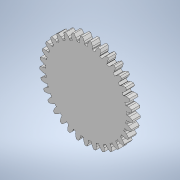
# Autodesk Inventor part: m1歯数33ギア3t
Saved by Autodesk Inventor 2020.2 (Build 242310000, 310)
## iProperties
Created: 2020-02-29
Part Number: m1歯数33ギア3t
Material: 一般
Document SubType Name: Modeling
Designer: aoyam
Density: 1 g/cm^3
Appearance: 既定
Author: aoyam
Autodesk Inventor part; units mm, degrees
ref_plane "YZ Plane" through (0, 0, 0) normal (1, 0, 0) x (0, 1, 0)
ref_plane "XZ Plane" through (0, 0, 0) normal (0, 1, 0) x (-1, 0, 0)
ref_plane "XY Plane" through (0, 0, 0) normal (0, 0, 1) x (1, 0, 0)
sketch "スケッチ1" plane through (0, 0, 0) normal (0, 0, 1) x (1, 0, 0)
  arc A0 (1.4847, 16.4043) -> (1.4561, 16.2027) centre (2.8638, 16.106) ccw
  arc A1 (1.672, 17.032) -> (1.4847, 16.4043) centre (5.2725, 15.6154) ccw
  arc A2 (2.2412, 18.1583) -> (1.672, 17.032) centre (7.8648, 14.6094) ccw
  arc A3 (0.4424, 16.2027) -> (0.4138, 16.4043) centre (-0.9654, 16.106) ccw
  arc A4 (0.4138, 16.4043) -> (0.2264, 17.032) centre (-3.3741, 15.6154) ccw
  arc A5 (0.2264, 17.032) -> (-0.3427, 18.1583) centre (-5.9663, 14.6094) ccw
  arc A6 (1.4478, 15.9479) -> (0.4507, 15.9479) centre (0.9492, 0.706) ccw
  arc A7 (-0.3427, 18.1583) -> (-1.085, 18.0874) centre (0.9492, 0.706) ccw
  line L0 (1.4478, 15.9479) -> (1.4561, 16.2027)
  line L1 (0.4507, 15.9479) -> (0.4424, 16.2027)
  arc A8 (-1.4959, 16.2219) -> (-1.4858, 16.0185) centre (-0.0852, 16.19) ccw
  arc A9 (-1.4458, 15.7668) -> (-2.4248, 15.5781) centre (0.9492, 0.706) ccw
  line L2 (-1.4458, 15.7668) -> (-1.4858, 16.0185)
  line L3 (-2.4248, 15.5781) -> (-2.4812, 15.8267)
  arc A10 (-2.4812, 15.8267) -> (-2.5474, 16.0192) centre (-3.8452, 15.4653) ccw
  arc A11 (-1.4307, 16.8737) -> (-1.4959, 16.2219) centre (2.3728, 16.1641) ccw
  arc A12 (-2.5474, 16.0192) -> (-2.8502, 16.6001) centre (-6.1176, 14.5278) ccw
  arc A13 (-3.6222, 17.5984) -> (-4.3377, 17.3883) centre (0.9492, 0.706) ccw
  arc A14 (-2.8502, 16.6001) -> (-3.6222, 17.5984) centre (-8.4726, 13.0493) ccw
  arc A15 (-1.085, 18.0874) -> (-1.4307, 16.8737) centre (5.1086, 15.6669) ccw
  arc A16 (-4.3881, 15.4788) -> (-4.3397, 15.281) centre (-2.9969, 15.7144) ccw
  arc A17 (-4.2528, 15.0414) -> (-5.1784, 14.6708) centre (0.9492, 0.706) ccw
  line L4 (-4.2528, 15.0414) -> (-4.3397, 15.281)
  line L5 (-5.1784, 14.6708) -> (-5.2808, 14.9042)
  arc A18 (-5.2808, 14.9042) -> (-5.3823, 15.0808) centre (-6.5518, 14.2913) ccw
  arc A19 (-4.4475, 16.1311) -> (-4.3881, 15.4788) centre (-0.5784, 16.1542) ccw
  arc A20 (-5.3823, 15.0808) -> (-5.7895, 15.5939) centre (-8.6056, 12.9406) ccw
  arc A21 (-6.7365, 16.4279) -> (-7.3993, 16.0863) centre (0.9492, 0.706) ccw
  arc A22 (-5.7895, 15.5939) -> (-6.7365, 16.4279) centre (-10.6383, 11.0432) ccw
  arc A23 (-4.3377, 17.3883) -> (-4.4475, 16.1311) centre (2.2021, 16.1837) ccw
  arc A24 (-7.0874, 14.2017) -> (-7.0025, 14.0167) centre (-5.7659, 14.6964) ccw
  arc A25 (-6.8717, 13.7978) -> (-7.7105, 13.2588) centre (0.9492, 0.706) ccw
  line L6 (-6.8717, 13.7978) -> (-7.0025, 14.0167)
  line L7 (-7.7105, 13.2588) -> (-7.8553, 13.4686)
  arc A26 (-7.8553, 13.4686) -> (-7.9883, 13.6227) centre (-8.9873, 12.6262) ccw
  arc A27 (-7.2692, 14.8311) -> (-7.0874, 14.2017) centre (-3.4744, 15.5859) ccw
  arc A28 (-7.9883, 13.6227) -> (-8.4853, 14.0495) centre (-10.7484, 10.9112) ccw
  arc A29 (-9.573, 14.6893) -> (-10.1591, 14.2284) centre (0.9492, 0.706) ccw
  arc A30 (-8.4853, 14.0495) -> (-9.573, 14.6893) centre (-12.3852, 8.6634) ccw
  arc A31 (-7.3993, 16.0863) -> (-7.2692, 14.8311) centre (-0.7497, 16.1411) ccw
  arc A32 (-9.4963, 12.4369) -> (-9.3778, 12.2712) centre (-8.2923, 13.1727) ccw
  arc A33 (-9.208, 12.0811) -> (-9.9296, 11.3931) centre (0.9492, 0.706) ccw
  line L8 (-9.208, 12.0811) -> (-9.3778, 12.2712)
  line L9 (-9.9296, 11.3931) -> (-10.1115, 11.5717)
  arc A34 (-10.1115, 11.5717) -> (-10.2713, 11.6979) centre (-11.0636, 10.5303) ccw
  arc A35 (-9.7938, 13.0204) -> (-9.4963, 12.4369) centre (-6.2105, 14.4799) ccw
  arc A36 (-10.2713, 11.6979) -> (-10.8401, 12.0229) centre (-12.4683, 8.513) ccw
  arc A37 (-12.0292, 12.4452) -> (-12.5175, 11.8817) centre (0.9492, 0.706) ccw
  arc A38 (-10.8401, 12.0229) -> (-12.0292, 12.4452) centre (-13.6502, 5.9961) ccw
  arc A39 (-10.1591, 14.2284) -> (-9.7938, 13.0204) centre (-3.6401, 15.5406) ccw
  arc A40 (-11.5276, 10.248) -> (-11.3799, 10.1078) centre (-10.4846, 11.1985) ccw
  arc A41 (-11.1772, 9.9532) -> (-11.7556, 9.1411) centre (0.9492, 0.706) ccw
  line L10 (-11.1772, 9.9532) -> (-11.3799, 10.1078)
  line L11 (-11.7556, 9.1411) -> (-11.968, 9.2821)
  arc A42 (-11.968, 9.2821) -> (-12.1487, 9.3758) centre (-12.7058, 8.0793) ccw
  arc A43 (-11.9302, 10.7648) -> (-11.5276, 10.248) centre (-8.6878, 12.876) ccw
  arc A44 (-12.1487, 9.3758) -> (-12.7687, 9.5872) centre (-13.7033, 5.8326) ccw
  arc A45 (-14.0164, 9.7769) -> (-14.3892, 9.1312) centre (0.9492, 0.706) ccw
  arc A46 (-12.7687, 9.5872) -> (-14.0164, 9.7769) centre (-14.3875, 3.1375) ccw
  arc A47 (-12.5175, 11.8817) -> (-11.9302, 10.7648) centre (-6.3647, 14.404) ccw
  arc A48 (-13.108, 7.7143) -> (-12.9364, 7.6046) centre (-12.2637, 8.845) ccw
  arc A49 (-12.7081, 7.4912) -> (-13.1223, 6.5843) centre (0.9492, 0.706) ccw
  line L12 (-12.7081, 7.4912) -> (-12.9364, 7.6046)
  line L13 (-13.1223, 6.5843) -> (-13.3576, 6.6825)
  arc A50 (-13.3576, 6.6825) -> (-13.5528, 6.7403) centre (-13.8544, 5.3618) ccw
  arc A51 (-13.6011, 8.1455) -> (-13.108, 7.7143) centre (-10.8168, 10.8322) ccw
  arc A52 (-13.5528, 6.7403) -> (-14.2016, 6.8306) centre (-14.4088, 2.967) ccw
  arc A53 (-15.4626, 6.7807) -> (-15.7065, 6.0761) centre (0.9492, 0.706) ccw
  arc A54 (-14.2016, 6.8306) -> (-15.4626, 6.7807) centre (-14.5705, 0.1911) ccw
  arc A55 (-14.3892, 9.1312) -> (-13.6011, 8.1455) centre (-8.8249, 12.7723) ccw
  arc A56 (-14.1803, 4.9274) -> (-13.9911, 4.8521) centre (-13.5652, 6.1973) ccw
  arc A57 (-13.7454, 4.7839) -> (-13.9805, 3.815) centre (0.9492, 0.706) ccw
  line L14 (-13.7454, 4.7839) -> (-13.9911, 4.8521)
  line L15 (-13.9805, 3.815) -> (-14.2301, 3.8669)
  arc A58 (-14.2301, 3.8669) -> (-14.4327, 3.8867) centre (-14.468, 2.4761) ccw
  arc A59 (-14.7461, 5.2574) -> (-14.1803, 4.9274) centre (-12.5206, 8.4225) ccw
  arc A60 (-14.4327, 3.8867) -> (-15.0869, 3.8526) centre (-14.5591, 0.0196) ccw
  arc A61 (-16.3156, 3.565) -> (-16.4218, 2.827) centre (0.9492, 0.706) ccw
  arc A62 (-15.0869, 3.8526) -> (-16.3156, 3.565) centre (-14.1926, -2.7368) ccw
  arc A63 (-15.7065, 6.0761) -> (-14.7461, 5.2574) centre (-10.9318, 10.7045) ccw
  arc A64 (-14.7057, 1.9878) -> (-14.5057, 1.9497) centre (-14.3422, 3.3512) ccw
  arc A65 (-14.2516, 1.9292) -> (-14.2991, 0.9333) centre (0.9492, 0.706) ccw
  line L16 (-14.2516, 1.9292) -> (-14.5057, 1.9497)
  line L17 (-14.2991, 0.9333) -> (-14.554, 0.9371)
  arc A66 (-14.554, 0.9371) -> (-14.7567, 0.9182) centre (-14.5244, -0.4736) ccw
  arc A67 (-15.3238, 2.2048) -> (-14.7057, 1.9878) centre (-13.7375, 5.7339) ccw
  arc A68 (-14.7567, 0.9182) -> (-15.3926, 0.7609) centre (-14.1489, -2.903) ccw
  arc A69 (-16.5447, 0.2459) -> (-16.5092, -0.4989) centre (0.9492, 0.706) ccw
  arc A70 (-15.3926, 0.7609) -> (-16.5447, 0.2459) centre (-13.2674, -5.5401) ccw
  arc A71 (-16.4218, 2.827) -> (-15.3238, 2.2048) centre (-12.6093, 8.2753) ccw
  arc A72 (-14.6654, -0.9981) -> (-14.4618, -0.9977) centre (-14.5664, 0.4095) ccw
  arc A73 (-14.2084, -0.9697) -> (-14.0665, -1.9566) centre (0.9492, 0.706) ccw
  line L18 (-14.2084, -0.9697) -> (-14.4618, -0.9977)
  line L19 (-14.0665, -1.9566) -> (-14.3175, -2.0011)
  arc A74 (-14.3175, -2.0011) -> (-14.513, -2.058) centre (-14.0215, -3.3807) ccw
  arc A75 (-15.3134, -0.902) -> (-14.6654, -0.9981) centre (-14.4236, 2.8635) ccw
  arc A76 (-14.513, -2.058) -> (-15.1077, -2.3328) centre (-13.1931, -5.6951) ccw
  arc A77 (-16.1415, -3.0565) -> (-15.9657, -3.7811) centre (0.9492, 0.706) ccw
  arc A78 (-15.1077, -2.3328) -> (-16.1415, -3.0565) centre (-11.8284, -8.1178) ccw
  arc A79 (-16.5092, -0.4989) -> (-15.3134, -0.902) centre (-13.7968, 5.5725) ccw
  arc A80 (-14.0607, -3.9224) -> (-13.8609, -3.8835) centre (-14.2299, -2.5215) ccw
  arc A81 (-13.6174, -3.808) -> (-13.2913, -4.7502) centre (0.9492, 0.706) ccw
  line L20 (-13.6174, -3.808) -> (-13.8609, -3.8835)
  line L21 (-13.2913, -4.7502) -> (-13.5293, -4.8414)
  arc A82 (-13.5293, -4.8414) -> (-13.7105, -4.9343) centre (-12.9775, -6.1401) ccw
  arc A83 (-14.7152, -3.9506) -> (-14.0607, -3.9224) centre (-14.5541, -0.0848) ccw
  arc A84 (-13.7105, -4.9343) -> (-14.2424, -5.3167) centre (-11.7261, -8.2559) ccw
  arc A85 (-15.1206, -6.223) -> (-14.8108, -6.9012) centre (0.9492, 0.706) ccw
  arc A86 (-14.2424, -5.3167) -> (-15.1206, -6.223) centre (-9.9276, -10.3765) ccw
  arc A87 (-15.9657, -3.7811) -> (-14.7152, -3.9506) centre (-14.4513, 2.6939) ccw
  arc A88 (-12.9135, -6.6794) -> (-12.7247, -6.6033) centre (-13.3448, -5.3359) ccw
  arc A89 (-12.4998, -6.4832) -> (-12.0013, -7.3466) centre (0.9492, 0.706) ccw
  line L22 (-12.4998, -6.4832) -> (-12.7247, -6.6033)
  line L23 (-12.0013, -7.3466) -> (-12.2178, -7.4812)
  arc A90 (-12.2178, -7.4812) -> (-12.3781, -7.6068) centre (-11.4302, -8.652) ccw
  arc A91 (-13.5508, -6.831) -> (-12.9135, -6.6794) centre (-14.1243, -3.0046) ccw
  arc A92 (-12.3781, -7.6068) -> (-12.828, -8.0829) centre (-9.801, -10.4928) ccw
  arc A93 (-13.5189, -9.139) -> (-13.0864, -9.7464) centre (0.9492, 0.706) ccw
  arc A94 (-12.828, -8.0829) -> (-13.5189, -9.139) centre (-7.6336, -12.2347) ccw
  arc A95 (-14.8108, -6.9012) -> (-13.5508, -6.831) centre (-14.5492, -0.2566) ccw
  arc A96 (-11.2653, -9.1695) -> (-11.0943, -9.0591) centre (-11.9431, -7.9319) ccw
  arc A97 (-10.8962, -8.8985) -> (-10.2433, -9.652) centre (0.9492, 0.706) ccw
  line L24 (-10.8962, -8.8985) -> (-11.0943, -9.0591)
  line L25 (-10.2433, -9.652) -> (-10.4304, -9.8252)
  arc A98 (-10.4304, -9.8252) -> (-10.5641, -9.9788) centre (-9.4355, -10.8258) ccw
  arc A99 (-11.8624, -9.4389) -> (-11.2653, -9.1695) centre (-13.1497, -5.7902) ccw
  arc A100 (-10.5641, -9.9788) -> (-10.9158, -10.5314) centre (-7.4873, -12.3249) ccw
  arc A101 (-11.3942, -11.6992) -> (-10.8546, -12.2137) centre (0.9492, 0.706) ccw
  arc A102 (-10.9158, -10.5314) -> (-11.3942, -11.6992) centre (-5.0295, -13.6252) ccw
  arc A103 (-13.0864, -9.7464) -> (-11.8624, -9.4389) centre (-14.0869, -3.1723) ccw
  arc A104 (-9.1756, -11.3026) -> (-9.0286, -11.1618) centre (-10.0754, -10.2156) ccw
  arc A105 (-8.8645, -10.9667) -> (-8.0808, -11.583) centre (0.9492, 0.706) ccw
  line L26 (-8.8645, -10.9667) -> (-9.0286, -11.1618)
  line L27 (-8.0808, -11.583) -> (-8.2317, -11.7885)
  arc A106 (-8.2317, -11.7885) -> (-8.3339, -11.9646) centre (-7.0654, -12.5827) ccw
  arc A107 (-9.7109, -11.6802) -> (-9.1756, -11.3026) centre (-11.6655, -8.341) ccw
  arc A108 (-8.3339, -11.9646) -> (-8.5746, -12.5738) centre (-4.8688, -13.686) ccw
  arc A109 (-8.8235, -13.811) -> (-8.1962, -14.2141) centre (0.9492, 0.706) ccw
  arc A110 (-8.5746, -12.5738) -> (-8.8235, -13.811) centre (-2.2092, -14.4977) ccw
  arc A111 (-10.8546, -12.2137) -> (-9.7109, -11.6802) centre (-13.0812, -5.9478) ccw
  arc A112 (-6.72, -13.0018) -> (-6.6022, -12.8357) centre (-7.8092, -12.1047) ccw
  arc A113 (-6.4781, -12.613) -> (-5.5919, -13.0699) centre (0.9492, 0.706) ccw
  line L28 (-6.4781, -12.613) -> (-6.6022, -12.8357)
  line L29 (-5.5919, -13.0699) -> (-5.7012, -13.3002)
  arc A114 (-5.7012, -13.3002) -> (-5.7682, -13.4925) centre (-4.4057, -13.8593) ccw
  arc A115 (-7.1742, -13.4738) -> (-6.72, -13.0018) centre (-9.7253, -10.5649) ccw
  arc A116 (-5.7682, -13.4925) -> (-5.8893, -14.1363) centre (-2.0399, -14.527) ccw
  arc A117 (-5.8995, -15.3982) -> (-5.2073, -15.6753) centre (0.9492, 0.706) ccw
  arc A118 (-5.8893, -14.1363) -> (-5.8995, -15.3982) centre (0.7251, -14.8207) ccw
  arc A119 (-8.1962, -14.2141) -> (-7.1742, -13.4738) centre (-11.5684, -8.4829) ccw
  arc A120 (-3.9872, -14.2055) -> (-3.903, -14.0201) centre (-5.2265, -13.5307) ccw
  arc A121 (-3.8232, -13.778) -> (-2.8666, -14.0589) centre (0.9492, 0.706) ccw
  line L30 (-3.8232, -13.778) -> (-3.903, -14.0201)
  line L31 (-2.8666, -14.0589) -> (-2.9303, -14.3057)
  arc A122 (-2.9303, -14.3057) -> (-2.9597, -14.5072) centre (-1.5524, -14.6095) ccw
  arc A123 (-4.3438, -14.755) -> (-3.9872, -14.2055) centre (-7.3994, -12.3814) ccw
  arc A124 (-2.9597, -14.5072) -> (-2.9568, -15.1622) centre (0.897, -14.8174) ccw
  arc A125 (-2.728, -16.4033) -> (-1.9958, -16.5444) centre (0.9492, 0.706) ccw
  arc A126 (-2.9568, -15.1622) -> (-2.728, -16.4033) centre (3.6676, -14.5825) ccw
  arc A127 (-5.2073, -15.6753) -> (-4.3438, -14.755) centre (-9.6032, -10.6858) ccw
  arc A128 (-1.076, -14.8702) -> (-1.0284, -14.6723) centre (-2.4205, -14.4422) ccw
  arc A129 (-0.9958, -14.4194) -> (-0.0033, -14.5142) centre (0.9492, 0.706) ccw
  line L32 (-0.9958, -14.4194) -> (-1.0284, -14.6723)
  line L33 (-0.0033, -14.5142) -> (-0.0193, -14.7686)
  arc A130 (-0.0193, -14.7686) -> (-0.01, -14.972) centre (1.3913, -14.8062) ccw
  arc A131 (-1.3222, -15.4773) -> (-1.076, -14.8702) centre (-4.7717, -13.7249) ccw
  arc A132 (-0.01, -14.972) -> (0.1169, -15.6147) centre (3.8357, -14.5468) ccw
  arc A133 (0.5764, -16.79) -> (1.3221, -16.79) centre (0.9492, 0.706) ccw
  arc A134 (0.1169, -15.6147) -> (0.5764, -16.79) centre (6.5119, -13.7917) ccw
  arc A135 (-1.9958, -16.5444) -> (-1.3222, -15.4773) centre (-7.2566, -12.477) ccw
  arc A136 (1.9085, -14.972) -> (1.9177, -14.7686) centre (0.5072, -14.8062) ccw
  arc A137 (1.9018, -14.5142) -> (2.8943, -14.4194) centre (0.9492, 0.706) ccw
  line L34 (1.9018, -14.5142) -> (1.9177, -14.7686)
  line L35 (2.8943, -14.4194) -> (2.9268, -14.6723)
  arc A138 (2.9268, -14.6723) -> (2.9744, -14.8702) centre (4.319, -14.4422) ccw
  arc A139 (1.7816, -15.6147) -> (1.9085, -14.972) centre (-1.9373, -14.5468) ccw
  arc A140 (2.9744, -14.8702) -> (3.2206, -15.4773) centre (6.6702, -13.7249) ccw
  arc A141 (3.8943, -16.5444) -> (4.6265, -16.4033) centre (0.9492, 0.706) ccw
  arc A142 (3.2206, -15.4773) -> (3.8943, -16.5444) centre (9.1551, -12.477) ccw
  arc A143 (1.3221, -16.79) -> (1.7816, -15.6147) centre (-4.6134, -13.7917) ccw
  arc A144 (4.8582, -14.5072) -> (4.8288, -14.3057) centre (3.4509, -14.6095) ccw
  arc A145 (4.765, -14.0589) -> (5.7217, -13.778) centre (0.9492, 0.706) ccw
  line L36 (4.765, -14.0589) -> (4.8288, -14.3057)
  line L37 (5.7217, -13.778) -> (5.8015, -14.0201)
  arc A146 (5.8015, -14.0201) -> (5.8857, -14.2055) centre (7.1249, -13.5307) ccw
  arc A147 (4.8553, -15.1622) -> (4.8582, -14.5072) centre (1.0015, -14.8174) ccw
  arc A148 (5.8857, -14.2055) -> (6.2423, -14.755) centre (9.2979, -12.3814) ccw
  arc A149 (7.1057, -15.6753) -> (7.798, -15.3982) centre (0.9492, 0.706) ccw
  arc A150 (6.2423, -14.755) -> (7.1057, -15.6753) centre (11.5017, -10.6858) ccw
  arc A151 (4.6265, -16.4033) -> (4.8553, -15.1622) centre (-1.7692, -14.5825) ccw
  arc A152 (7.6667, -13.4925) -> (7.5997, -13.3002) centre (6.3042, -13.8593) ccw
  arc A153 (7.4904, -13.0699) -> (8.3766, -12.613) centre (0.9492, 0.706) ccw
  line L38 (7.4904, -13.0699) -> (7.5997, -13.3002)
  line L39 (8.3766, -12.613) -> (8.5007, -12.8357)
  arc A154 (8.5007, -12.8357) -> (8.6185, -13.0018) centre (9.7077, -12.1047) ccw
  arc A155 (7.7878, -14.1363) -> (7.6667, -13.4925) centre (3.9384, -14.527) ccw
  arc A156 (8.6185, -13.0018) -> (9.0727, -13.4738) centre (11.6238, -10.5649) ccw
  arc A157 (10.0947, -14.2141) -> (10.7219, -13.811) centre (0.9492, 0.706) ccw
  arc A158 (9.0727, -13.4738) -> (10.0947, -14.2141) centre (13.4669, -8.4829) ccw
  arc A159 (7.798, -15.3982) -> (7.7878, -14.1363) centre (1.1733, -14.8207) ccw
  arc A160 (10.2324, -11.9646) -> (10.1302, -11.7885) centre (8.9639, -12.5827) ccw
  arc A161 (9.9793, -11.583) -> (10.763, -10.9667) centre (0.9492, 0.706) ccw
  line L40 (9.9793, -11.583) -> (10.1302, -11.7885)
  line L41 (10.763, -10.9667) -> (10.927, -11.1618)
  arc A162 (10.927, -11.1618) -> (11.0741, -11.3026) centre (11.9738, -10.2156) ccw
  arc A163 (10.4731, -12.5738) -> (10.2324, -11.9646) centre (6.7672, -13.686) ccw
  arc A164 (11.0741, -11.3026) -> (11.6094, -11.6802) centre (13.5639, -8.341) ccw
  arc A165 (12.7531, -12.2137) -> (13.2927, -11.6992) centre (0.9492, 0.706) ccw
  arc A166 (11.6094, -11.6802) -> (12.7531, -12.2137) centre (14.9797, -5.9478) ccw
  arc A167 (10.7219, -13.811) -> (10.4731, -12.5738) centre (4.1077, -14.4977) ccw
  arc A168 (12.4625, -9.9788) -> (12.3289, -9.8252) centre (11.334, -10.8258) ccw
  arc A169 (12.1418, -9.652) -> (12.7947, -8.8985) centre (0.9492, 0.706) ccw
  line L42 (12.1418, -9.652) -> (12.3289, -9.8252)
  line L43 (12.7947, -8.8985) -> (12.9927, -9.0591)
  arc A170 (12.9927, -9.0591) -> (13.1638, -9.1695) centre (13.8415, -7.9319) ccw
  arc A171 (12.8142, -10.5314) -> (12.4625, -9.9788) centre (9.3858, -12.3249) ccw
  arc A172 (13.1638, -9.1695) -> (13.7609, -9.4389) centre (15.0482, -5.7902) ccw
  arc A173 (14.9848, -9.7464) -> (15.4173, -9.139) centre (0.9492, 0.706) ccw
  arc A174 (13.7609, -9.4389) -> (14.9848, -9.7464) centre (15.9854, -3.1723) ccw
  arc A175 (13.2927, -11.6992) -> (12.8142, -10.5314) centre (6.928, -13.6252) ccw
  arc A176 (14.2766, -7.6068) -> (14.1163, -7.4812) centre (13.3287, -8.652) ccw
  arc A177 (13.8998, -7.3466) -> (14.3983, -6.4832) centre (0.9492, 0.706) ccw
  line L44 (13.8998, -7.3466) -> (14.1163, -7.4812)
  line L45 (14.3983, -6.4832) -> (14.6232, -6.6033)
  arc A178 (14.6232, -6.6033) -> (14.812, -6.6794) centre (15.2433, -5.3359) ccw
  arc A179 (14.7265, -8.0829) -> (14.2766, -7.6068) centre (11.6995, -10.4928) ccw
  arc A180 (14.812, -6.6794) -> (15.4493, -6.831) centre (16.0228, -3.0046) ccw
  arc A181 (16.7093, -6.9012) -> (17.0191, -6.223) centre (0.9492, 0.706) ccw
  arc A182 (15.4493, -6.831) -> (16.7093, -6.9012) centre (16.4477, -0.2566) ccw
  arc A183 (15.4173, -9.139) -> (14.7265, -8.0829) centre (9.5321, -12.2347) ccw
  arc A184 (15.609, -4.9343) -> (15.4278, -4.8414) centre (14.876, -6.1401) ccw
  arc A185 (15.1898, -4.7502) -> (15.5158, -3.808) centre (0.9492, 0.706) ccw
  line L46 (15.1898, -4.7502) -> (15.4278, -4.8414)
  line L47 (15.5158, -3.808) -> (15.7594, -3.8835)
  arc A186 (15.7594, -3.8835) -> (15.9592, -3.9224) centre (16.1284, -2.5215) ccw
  arc A187 (16.1409, -5.3167) -> (15.609, -4.9343) centre (13.6246, -8.2559) ccw
  arc A188 (15.9592, -3.9224) -> (16.6137, -3.9506) centre (16.4526, -0.0848) ccw
  arc A189 (17.8642, -3.7811) -> (18.04, -3.0565) centre (0.9492, 0.706) ccw
  arc A190 (16.6137, -3.9506) -> (17.8642, -3.7811) centre (16.3498, 2.6939) ccw
  arc A191 (17.0191, -6.223) -> (16.1409, -5.3167) centre (11.8261, -10.3765) ccw
  arc A192 (16.4115, -2.058) -> (16.216, -2.0011) centre (15.92, -3.3807) ccw
  arc A193 (15.965, -1.9566) -> (16.1069, -0.9697) centre (0.9492, 0.706) ccw
  line L48 (15.965, -1.9566) -> (16.216, -2.0011)
  line L49 (16.1069, -0.9697) -> (16.3603, -0.9977)
  arc A194 (16.3603, -0.9977) -> (16.5639, -0.9981) centre (16.4649, 0.4095) ccw
  arc A195 (17.0061, -2.3328) -> (16.4115, -2.058) centre (15.0916, -5.6951) ccw
  arc A196 (16.5639, -0.9981) -> (17.2119, -0.902) centre (16.3221, 2.8635) ccw
  arc A197 (18.4077, -0.4989) -> (18.4432, 0.2459) centre (0.9492, 0.706) ccw
  arc A198 (17.2119, -0.902) -> (18.4077, -0.4989) centre (15.6953, 5.5725) ccw
  arc A199 (18.04, -3.0565) -> (17.0061, -2.3328) centre (13.7269, -8.1178) ccw
  arc A200 (16.6552, 0.9182) -> (16.4524, 0.9371) centre (16.4229, -0.4736) ccw
  arc A201 (16.1975, 0.9333) -> (16.1501, 1.9292) centre (0.9492, 0.706) ccw
  line L50 (16.1975, 0.9333) -> (16.4524, 0.9371)
  line L51 (16.1501, 1.9292) -> (16.4042, 1.9497)
  arc A202 (16.4042, 1.9497) -> (16.6042, 1.9878) centre (16.2407, 3.3512) ccw
  arc A203 (17.2911, 0.7609) -> (16.6552, 0.9182) centre (16.0474, -2.903) ccw
  arc A204 (16.6042, 1.9878) -> (17.2223, 2.2048) centre (15.636, 5.7339) ccw
  arc A205 (18.3202, 2.827) -> (18.2141, 3.565) centre (0.9492, 0.706) ccw
  arc A206 (17.2223, 2.2048) -> (18.3202, 2.827) centre (14.5078, 8.2753) ccw
  arc A207 (18.4432, 0.2459) -> (17.2911, 0.7609) centre (15.1659, -5.5401) ccw
  arc A208 (16.3312, 3.8867) -> (16.1286, 3.8669) centre (16.3665, 2.4761) ccw
  arc A209 (15.879, 3.815) -> (15.6439, 4.7839) centre (0.9492, 0.706) ccw
  line L52 (15.879, 3.815) -> (16.1286, 3.8669)
  line L53 (15.6439, 4.7839) -> (15.8896, 4.8521)
  arc A210 (15.8896, 4.8521) -> (16.0787, 4.9274) centre (15.4637, 6.1973) ccw
  arc A211 (16.9854, 3.8526) -> (16.3312, 3.8867) centre (16.4576, 0.0196) ccw
  arc A212 (16.0787, 4.9274) -> (16.6446, 5.2574) centre (14.4191, 8.4225) ccw
  arc A213 (17.6049, 6.0761) -> (17.3611, 6.7807) centre (0.9492, 0.706) ccw
  arc A214 (16.6446, 5.2574) -> (17.6049, 6.0761) centre (12.8303, 10.7045) ccw
  arc A215 (18.2141, 3.565) -> (16.9854, 3.8526) centre (16.0911, -2.7368) ccw
  arc A216 (15.4513, 6.7403) -> (15.256, 6.6825) centre (15.7529, 5.3618) ccw
  arc A217 (15.0208, 6.5843) -> (14.6066, 7.4912) centre (0.9492, 0.706) ccw
  line L54 (15.0208, 6.5843) -> (15.256, 6.6825)
  line L55 (14.6066, 7.4912) -> (14.8349, 7.6046)
  arc A218 (14.8349, 7.6046) -> (15.0064, 7.7143) centre (14.1622, 8.845) ccw
  arc A219 (16.1001, 6.8306) -> (15.4513, 6.7403) centre (16.3072, 2.967) ccw
  arc A220 (15.0064, 7.7143) -> (15.4996, 8.1455) centre (12.7153, 10.8322) ccw
  arc A221 (16.2877, 9.1312) -> (15.9148, 9.7769) centre (0.9492, 0.706) ccw
  arc A222 (15.4996, 8.1455) -> (16.2877, 9.1312) centre (10.7233, 12.7723) ccw
  arc A223 (17.3611, 6.7807) -> (16.1001, 6.8306) centre (16.469, 0.1911) ccw
  arc A224 (14.0472, 9.3758) -> (13.8664, 9.2821) centre (14.6042, 8.0793) ccw
  arc A225 (13.6541, 9.1411) -> (13.0757, 9.9532) centre (0.9492, 0.706) ccw
  line L56 (13.6541, 9.1411) -> (13.8664, 9.2821)
  line L57 (13.0757, 9.9532) -> (13.2784, 10.1078)
  arc A226 (13.2784, 10.1078) -> (13.4261, 10.248) centre (12.3831, 11.1985) ccw
  arc A227 (14.6672, 9.5872) -> (14.0472, 9.3758) centre (15.6018, 5.8326) ccw
  arc A228 (13.4261, 10.248) -> (13.8287, 10.7648) centre (10.5863, 12.876) ccw
  arc A229 (14.416, 11.8817) -> (13.9277, 12.4452) centre (0.9492, 0.706) ccw
  arc A230 (13.8287, 10.7648) -> (14.416, 11.8817) centre (8.2632, 14.404) ccw
  arc A231 (15.9148, 9.7769) -> (14.6672, 9.5872) centre (16.286, 3.1375) ccw
  arc A232 (12.1698, 11.6979) -> (12.01, 11.5717) centre (12.9621, 10.5303) ccw
  arc A233 (11.8281, 11.3931) -> (11.1065, 12.0811) centre (0.9492, 0.706) ccw
  line L58 (11.8281, 11.3931) -> (12.01, 11.5717)
  line L59 (11.1065, 12.0811) -> (11.2763, 12.2712)
  arc A234 (11.2763, 12.2712) -> (11.3948, 12.4369) centre (10.1908, 13.1727) ccw
  arc A235 (12.7385, 12.0229) -> (12.1698, 11.6979) centre (14.3668, 8.513) ccw
  arc A236 (11.3948, 12.4369) -> (11.6923, 13.0204) centre (8.109, 14.4799) ccw
  arc A237 (12.0576, 14.2284) -> (11.4715, 14.6893) centre (0.9492, 0.706) ccw
  arc A238 (11.6923, 13.0204) -> (12.0576, 14.2284) centre (5.5386, 15.5406) ccw
  arc A239 (13.9277, 12.4452) -> (12.7385, 12.0229) centre (15.5487, 5.9961) ccw
  arc A240 (9.8868, 13.6227) -> (9.7537, 13.4686) centre (10.8857, 12.6262) ccw
  arc A241 (9.609, 13.2588) -> (8.7702, 13.7978) centre (0.9492, 0.706) ccw
  line L60 (9.609, 13.2588) -> (9.7537, 13.4686)
  line L61 (8.7702, 13.7978) -> (8.901, 14.0167)
  arc A242 (8.901, 14.0167) -> (8.9859, 14.2017) centre (7.6644, 14.6964) ccw
  arc A243 (10.3838, 14.0495) -> (9.8868, 13.6227) centre (12.6468, 10.9112) ccw
  arc A244 (8.9859, 14.2017) -> (9.1677, 14.8311) centre (5.3729, 15.5859) ccw
  arc A245 (9.2978, 16.0863) -> (8.635, 16.4279) centre (0.9492, 0.706) ccw
  arc A246 (9.1677, 14.8311) -> (9.2978, 16.0863) centre (2.6482, 16.1411) ccw
  arc A247 (11.4715, 14.6893) -> (10.3838, 14.0495) centre (14.2837, 8.6634) ccw
  arc A248 (7.2807, 15.0808) -> (7.1793, 14.9042) centre (8.4503, 14.2913) ccw
  arc A249 (7.0769, 14.6708) -> (6.1513, 15.0414) centre (0.9492, 0.706) ccw
  line L62 (7.0769, 14.6708) -> (7.1793, 14.9042)
  line L63 (6.1513, 15.0414) -> (6.2382, 15.281)
  arc A250 (6.2382, 15.281) -> (6.2866, 15.4788) centre (4.8954, 15.7144) ccw
  arc A251 (7.688, 15.5939) -> (7.2807, 15.0808) centre (10.5041, 12.9406) ccw
  arc A252 (6.2866, 15.4788) -> (6.346, 16.1311) centre (2.4769, 16.1542) ccw
  arc A253 (6.2362, 17.3883) -> (5.5207, 17.5984) centre (0.9492, 0.706) ccw
  arc A254 (6.346, 16.1311) -> (6.2362, 17.3883) centre (-0.3036, 16.1837) ccw
  arc A255 (8.635, 16.4279) -> (7.688, 15.5939) centre (12.5368, 11.0432) ccw
  arc A256 (4.4459, 16.0192) -> (4.3797, 15.8267) centre (5.7437, 15.4653) ccw
  arc A257 (4.3233, 15.5781) -> (3.3443, 15.7668) centre (0.9492, 0.706) ccw
  line L64 (4.3233, 15.5781) -> (4.3797, 15.8267)
  line L65 (3.3443, 15.7668) -> (3.3843, 16.0185)
  arc A258 (3.3843, 16.0185) -> (3.3944, 16.2219) centre (1.9837, 16.19) ccw
  arc A259 (4.7487, 16.6001) -> (4.4459, 16.0192) centre (8.016, 14.5278) ccw
  arc A260 (3.3944, 16.2219) -> (3.3292, 16.8737) centre (-0.4743, 16.1641) ccw
  arc A261 (2.9835, 18.0874) -> (2.2412, 18.1583) centre (0.9492, 0.706) ccw
  arc A262 (3.3292, 16.8737) -> (2.9835, 18.0874) centre (-3.2101, 15.6669) ccw
  arc A263 (5.5207, 17.5984) -> (4.7487, 16.6001) centre (10.371, 13.0493) ccw
  point P0 (0, 0)
  point P1 (1.4478, 15.9479)
  point P2 (0.4507, 15.9479)
  point P3 (0.4138, 16.4043)
  point P4 (0.2264, 17.032)
  point P5 (-0.3427, 18.1583)
  point P6 (-1.085, 18.0874)
  point P7 (-1.4307, 16.8737)
  point P8 (-1.4959, 16.2219)
  point P9 (-1.4858, 16.0185)
  point P10 (-2.5474, 16.0192)
  point P11 (-2.8502, 16.6001)
  point P12 (-3.6222, 17.5984)
  point P13 (-4.3377, 17.3883)
  point P14 (-4.4475, 16.1311)
  point P15 (-4.3881, 15.4788)
  point P16 (-5.1784, 14.6708)
  point P17 (-5.3823, 15.0808)
  point P18 (-5.7895, 15.5939)
  point P19 (-6.7365, 16.4279)
  point P20 (-7.3993, 16.0863)
  point P21 (-7.2692, 14.8311)
  point P22 (-7.0874, 14.2017)
  point P23 (-7.9883, 13.6227)
  point P24 (-8.4853, 14.0495)
  point P25 (-9.573, 14.6893)
  point P26 (-10.1591, 14.2284)
  point P27 (-9.7938, 13.0204)
  point P28 (-9.4963, 12.4369)
  point P29 (-9.3778, 12.2712)
  point P30 (-9.9296, 11.3931)
  point P31 (-10.2713, 11.6979)
  point P32 (-12.0292, 12.4452)
  point P33 (-12.5175, 11.8817)
  point P34 (-11.9302, 10.7648)
  point P35 (-11.5276, 10.248)
  point P36 (-11.3799, 10.1078)
  point P37 (-11.968, 9.2821)
  point P38 (-12.7687, 9.5872)
  point P39 (-14.0164, 9.7769)
  point P40 (-14.3892, 9.1312)
  point P41 (-13.6011, 8.1455)
  point P42 (-13.108, 7.7143)
  point P43 (-12.9364, 7.6046)
  point P44 (-12.7081, 7.4912)
  point P45 (-13.3576, 6.6825)
  point P46 (-14.2016, 6.8306)
  point P47 (-15.7065, 6.0761)
  point P48 (-14.7461, 5.2574)
  point P49 (-14.1803, 4.9274)
  point P50 (-13.9805, 3.815)
  point P51 (-14.2301, 3.8669)
  point P52 (-14.4327, 3.8867)
  point P53 (-15.0869, 3.8526)
  point P54 (-16.3156, 3.565)
  point P55 (-16.4218, 2.827)
  point P56 (-15.3238, 2.2048)
  point P57 (-14.7057, 1.9878)
  point P58 (-14.5057, 1.9497)
  point P59 (-14.554, 0.9371)
  point P60 (-14.7567, 0.9182)
  point P61 (-15.3926, 0.7609)
  point P62 (-16.5447, 0.2459)
  point P63 (-16.5092, -0.4989)
  point P64 (-15.3134, -0.902)
  point P65 (-14.6654, -0.9981)
  point P66 (-14.513, -2.058)
  point P67 (-15.1077, -2.3328)
  point P68 (-16.1415, -3.0565)
  point P69 (-15.9657, -3.7811)
  point P70 (-14.7152, -3.9506)
  point P71 (-14.0607, -3.9224)
  point P72 (-13.6174, -3.808)
  point P73 (-13.2913, -4.7502)
  point P74 (-13.5293, -4.8414)
  point P75 (-13.7105, -4.9343)
  point P76 (-14.2424, -5.3167)
  point P77 (-15.1206, -6.223)
  point P78 (-14.8108, -6.9012)
  point P79 (-13.5508, -6.831)
  point P80 (-12.9135, -6.6794)
  point P81 (-12.3781, -7.6068)
  point P82 (-12.828, -8.0829)
  point P83 (-13.5189, -9.139)
  point P84 (-13.0864, -9.7464)
  point P85 (-11.8624, -9.4389)
  point P86 (-10.5641, -9.9788)
  point P87 (-10.9158, -10.5314)
  point P88 (-11.3942, -11.6992)
  point P89 (-10.8546, -12.2137)
  point P90 (-9.7109, -11.6802)
  point P91 (-9.1756, -11.3026)
  point P92 (-9.0286, -11.1618)
  point P93 (-8.8645, -10.9667)
  point P94 (-8.0808, -11.583)
  point P95 (-8.2317, -11.7885)
  point P96 (-8.3339, -11.9646)
  point P97 (-8.8235, -13.811)
  point P98 (-8.1962, -14.2141)
  point P99 (-7.1742, -13.4738)
  point P100 (-6.72, -13.0018)
  point P101 (-6.6022, -12.8357)
  point P102 (-6.4781, -12.613)
  point P103 (-5.5919, -13.0699)
  point P104 (-5.7012, -13.3002)
  point P105 (-5.7682, -13.4925)
  point P106 (-5.8893, -14.1363)
  point P107 (-5.8995, -15.3982)
  point P108 (-5.2073, -15.6753)
  point P109 (-4.3438, -14.755)
  point P110 (-3.9872, -14.2055)
  point P111 (-3.903, -14.0201)
  point P112 (-2.9597, -14.5072)
  point P113 (-2.9568, -15.1622)
  point P114 (-2.728, -16.4033)
  point P115 (-1.9958, -16.5444)
  point P116 (-1.3222, -15.4773)
  point P117 (-1.076, -14.8702)
  point P118 (-0.9958, -14.4194)
  point P119 (-0.01, -14.972)
  point P120 (0.1169, -15.6147)
  point P121 (0.5764, -16.79)
  point P122 (1.3221, -16.79)
  point P123 (1.7816, -15.6147)
  point P124 (1.9085, -14.972)
  point P125 (1.9018, -14.5142)
  point P126 (2.9744, -14.8702)
  point P127 (3.2206, -15.4773)
  point P128 (3.8943, -16.5444)
  point P129 (4.6265, -16.4033)
  point P130 (4.8553, -15.1622)
  point P131 (4.8582, -14.5072)
  point P132 (4.8288, -14.3057)
  point P133 (4.765, -14.0589)
  point P134 (5.7217, -13.778)
  point P135 (5.8015, -14.0201)
  point P136 (5.8857, -14.2055)
  point P137 (6.2423, -14.755)
  point P138 (7.1057, -15.6753)
  point P139 (7.798, -15.3982)
  point P140 (7.7878, -14.1363)
  point P141 (7.6667, -13.4925)
  point P142 (7.5997, -13.3002)
  point P143 (8.6185, -13.0018)
  point P144 (9.0727, -13.4738)
  point P145 (10.0947, -14.2141)
  point P146 (10.7219, -13.811)
  point P147 (10.4731, -12.5738)
  point P148 (10.2324, -11.9646)
  point P149 (10.1302, -11.7885)
  point P150 (9.9793, -11.583)
  point P151 (11.0741, -11.3026)
  point P152 (11.6094, -11.6802)
  point P153 (12.7531, -12.2137)
  point P154 (13.2927, -11.6992)
  point P155 (12.8142, -10.5314)
  point P156 (12.4625, -9.9788)
  point P157 (12.3289, -9.8252)
  point P158 (12.1418, -9.652)
  point P159 (13.1638, -9.1695)
  point P160 (13.7609, -9.4389)
  point P161 (14.9848, -9.7464)
  point P162 (15.4173, -9.139)
  point P163 (14.7265, -8.0829)
  point P164 (14.2766, -7.6068)
  point P165 (14.812, -6.6794)
  point P166 (15.4493, -6.831)
  point P167 (16.7093, -6.9012)
  point P168 (17.0191, -6.223)
  point P169 (16.1409, -5.3167)
  point P170 (15.609, -4.9343)
  point P171 (15.4278, -4.8414)
  point P172 (15.7594, -3.8835)
  point P173 (16.6137, -3.9506)
  point P174 (17.8642, -3.7811)
  point P175 (18.04, -3.0565)
  point P176 (17.0061, -2.3328)
  point P177 (16.4115, -2.058)
  point P178 (16.216, -2.0011)
  point P179 (16.3603, -0.9977)
  point P180 (16.5639, -0.9981)
  point P181 (17.2119, -0.902)
  point P182 (18.4077, -0.4989)
  point P183 (18.4432, 0.2459)
  point P184 (17.2911, 0.7609)
  point P185 (16.6552, 0.9182)
  point P186 (16.4524, 0.9371)
  point P187 (16.1975, 0.9333)
  point P188 (16.4042, 1.9497)
  point P189 (16.6042, 1.9878)
  point P190 (17.2223, 2.2048)
  point P191 (18.3202, 2.827)
  point P192 (18.2141, 3.565)
  point P193 (16.9854, 3.8526)
  point P194 (16.3312, 3.8867)
  point P195 (16.1286, 3.8669)
  point P196 (16.0787, 4.9274)
  point P197 (16.6446, 5.2574)
  point P198 (17.6049, 6.0761)
  point P199 (17.3611, 6.7807)
  dimension "d2" = 360
  constraints: 528 point on circle, 264 centre point, 132 end point, 2 coincident, 1253 other
extrude "押し出し1" add sketch "スケッチ1" along normal blind 3
